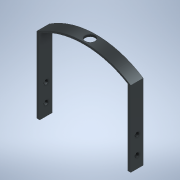
# Autodesk Inventor part: pulleybracket
Saved by Autodesk Inventor 2021.5 (Build 255421000, 421)
## iProperties
Created: 2024-11-18
Part Number: pulleybracket
Material: Iron, Cast
Document SubType Name: Modeling
Designer: email
Density: 7.15 g/cm^3
Appearance: Iron Gray
Author: email
Autodesk Inventor part; units mm, degrees
ref_plane "YZ Plane" through (0, 0, 0) normal (1, 0, 0) x (0, 1, 0)
ref_plane "XZ Plane" through (0, 0, 0) normal (0, 1, 0) x (-1, 0, 0)
sketch "Sketch1" plane through (0, 0, 0) normal (0, 0, 1) x (1, 0, 0)
  line L0 (0, 0) -> (88.9, 0)
  line L1 (0, 0) -> (-0.8653, 0)
  line L2 (88.9, 0) -> (18.4478, 0)
  line L3 (88.9, 22.8434) -> (88.9, 0)
  line L4 (0, 0) -> (-3, 0)
  line L5 (-3, 0) -> (-3, 76.2)
  line L6 (-3, 76.2) -> (0, 76.2)
  line L7 (0, 76.2) -> (0, 0)
  line L8 (88.9, 0) -> (91.9, 0)
  line L9 (91.9, 0) -> (91.9, 76.2)
  line L10 (91.9, 76.2) -> (88.9, 76.2)
  line L11 (88.9, 76.2) -> (88.9, 0)
  arc A0 (88.9, 76.2) -> (0, 76.2) centre (44.45, 1.8166) ccw
  arc A1 (91.9, 76.2) -> (-3, 76.2) centre (44.45, 4.8166) ccw
  dimension "d8" = 3
  dimension "d9" = 76.2
  dimension "d10" = 88.9
  dimension "d11" = 3
  dimension "d12" = 3
  constraints: 24 end point, 5 horizontal, 4 parallel, 4 point on circle, 2 centre point, 2 perpendicular
  measures "d8" distance between parallel lines of L7 L5
  measures "d9" distance of L4.end L5.end
  measures "d10" distance of L0.start L0.end
  measures "d11" distance between parallel lines of L9 L11
  measures "d12" distance of A1.centre A0.centre
extrude "Extrusion1" add sketch "Sketch1" along normal blind 12.6 contours L1 L4 L5 L6 L7 | L6 A1 L10 A0 | L3 L11 L10 L9 L8
sketch "Sketch2" plane through (91.9, 0, 0) normal (1, 0, 0) x (0, 0, -1)
  line L0 (0, 0) -> (-6.3, 0)
  line L1 (-6.3, 0) -> (-6.3, 30)
  line L2 (-6.3, 30) -> (0, 30)
  line L3 (0, 30) -> (0, 0)
  circle A0 centre (-6.3, 30) radius 2.35
  circle A1 centre (-6.3, 12) radius 2.35
  dimension "d15" = 30
  dimension "d16" = 6.3
  dimension "d17" = 4.7
  dimension "d18" = 4.7
  dimension "d19" = 18
  dimension "d26" = 12
  constraints: 8 end point, 2 centre point, 2 parallel, 1 coincident, 1 horizontal, 1 perpendicular, 1 point on line
  measures "d15" distance of L0.end L1.end
  measures "d16" distance of L1.end L2.end
  measures "d17" diameter of A0
  measures "d18" diameter of A1
  measures "d19" distance of A1.centre A0.centre
  measures "d26" distance from line of A1.centre L0
extrude "Extrusion2" cut sketch "Sketch2" against normal through all contours A1 L1 | L1 A1 | A0 L1 L2 | L2 L1 A0
ref_plane "Work Plane1" through (44.45, -80.8985, 0) normal (0, -1, 0) x (1, 0, 0)
sketch "Sketch3" plane through (44.45, -80.8985, 0) normal (0, -1, 0) x (1, 0, 0)
  line L0 (47.45, 0) -> (-47.45, 0) projected
  line L1 (-47.45, 0) -> (0, 0)
  line L2 (0, 0) -> (0, 6.3)
  line L3 (0, 6.3) -> (-47.45, 6.3)
  line L4 (-47.45, 6.3) -> (-47.45, 0)
  circle A0 centre (0, 6.3) radius 5
  point P0 (-44.45, 0)
  dimension "d22" = 6.3
  dimension "d23" = 10
  constraints: 8 end point, 2 parallel, 1 centre point, 1 coincident, 1 horizontal, 1 perpendicular
  measures "d22" distance of L1.end L2.end
  measures "d23" diameter of A0
extrude "Extrusion3" cut sketch "Sketch3" against normal through all contours A0 L3 L2 | L2 L3 A0
body "Solid1"
